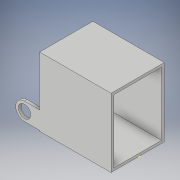
# Autodesk Inventor part: Tape measure holder case Albert
Saved by Autodesk Inventor 2019 (Build 230136000, 136)
## iProperties
Created: 2018-11-07
Part Number: Tape measure holder case Albert
Material: Generic
Document SubType Name: Modeling
Designer: mrhftc
Density: 1 g/cm^3
Appearance: Default
Author: mrhftc
Autodesk Inventor part; units mm, degrees
ref_plane "YZ Plane" through (0, 0, 0) normal (1, 0, 0) x (0, 1, 0)
ref_plane "XZ Plane" through (0, 0, 0) normal (0, 1, 0) x (-1, 0, 0)
ref_plane "XY Plane" through (0, 0, 0) normal (0, 0, 1) x (1, 0, 0)
sketch "Sketch1" plane through (0, 0, 0) normal (0, 1, 0) x (-1, 0, 0)
  line L0 (11.9219, 31.3255) -> (-68.5781, 31.3255)
  line L1 (-68.5781, 31.3255) -> (-68.5781, -28.6745)
  line L2 (-68.5781, -28.6745) -> (11.9219, -28.6745)
  line L3 (11.9219, -28.6745) -> (11.9219, 31.3255)
  point P0 (0, 0)
  dimension "d0" = 60
  dimension "d1" = 80.5
  constraints: 8 end point, 2 parallel, 1 horizontal, 1 perpendicular
  measures "d0" distance of L2.end L0.start
  measures "d1" distance of L0.start L0.end
extrude "Extrusion1" add sketch "Sketch1" along normal blind 77.4
sketch "Sketch2" plane through (68.5781, 0, 31.3255) normal (1, 0, 0) x (0, 0, -1)
  line L0 (3, 74.4) -> (57, 74.4)
  line L1 (57, 74.4) -> (57, 3)
  line L2 (57, 3) -> (3, 3)
  line L3 (3, 3) -> (3, 74.4)
  line L4 (0, 77.4) -> (60, 77.4) projected
  line L5 (0, 0) -> (0, 77.4) projected
  point P0 (31.3255, 0)
  dimension "d4" = 54
  dimension "d5" = 71.4
  dimension "d6" = 3
  dimension "d7" = 3
  constraints: 8 end point, 2 parallel, 1 horizontal, 1 perpendicular
  measures "d4" distance of L0.start L0.end
  measures "d5" distance of L0.end L1.end
  measures "d6" distance between parallel lines of L4 L0
  measures "d7" distance between parallel lines of L5 L3
sketch "Sketch3" plane through (68.5781, 0, 31.3255) normal (1, 0, 0) x (0, 0, -1)
  point P0 (31.3255, 0)
extrude "Extrusion2" cut sketch "Sketch2" against normal blind 74.5
sketch "Sketch4" plane through (-11.9219, 0, 31.3255) normal (0, 0, 1) x (1, 0, 0)
  line L0 (0, 1) -> (-17, 1)
  line L1 (-17, 21) -> (0, 21)
  line L2 (0, 21) -> (0, 1)
  line L3 (0, 0) -> (0, 77.4) projected
  line L4 (0, 0) -> (80.5, 0) projected
  circle A0 centre (-17, 11) radius 7
  arc A1 (-17, 21) -> (-17, 1) centre (-17, 11) ccw
  point P0 (11.9219, 0)
  dimension "d11" = 20
  dimension "d12" = 0
  dimension "d17" = 14
  dimension "d18" = 11
  dimension "d19" = 20
  dimension "d20" = 17
  constraints: 6 end point, 2 centre point, 2 point on circle, 1 coincident, 1 horizontal, 1 parallel
  measures "d11" distance of L1.end L0.start
  measures "d12" distance between parallel lines of L3 L2
  measures "d17" diameter of A0
  measures "d18" distance from line of L4 A0.centre
  measures "d19" diameter of A1
  measures "d20" distance from line of L2 A0.centre
extrude "Extrusion4" add sketch "Sketch4" against normal blind 3
body "Solid1"
